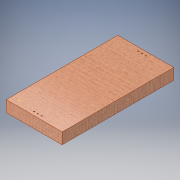
# Autodesk Inventor part: nhk19
Saved by Autodesk Inventor 2019 (Build 230136000, 136)
## iProperties
Created: 2022-02-15
Part Number: nhk19
Material: 木材 (オーク)
Document SubType Name: Sheet Metal
Designer: yuta
Density: 0.76 g/cm^3
Sheet Metal Rule: Default_mm
Appearance: ホワイト オーク材 - ナチュラル 標準の光沢
Author: yuta
Autodesk Inventor part; units mm, degrees
ref_plane "YZ Plane" through (0, 0, 0) normal (1, 0, 0) x (0, 1, 0)
ref_plane "XZ Plane" through (0, 0, 0) normal (0, 1, 0) x (-1, 0, 0)
ref_plane "XY Plane" through (0, 0, 0) normal (0, 0, 1) x (1, 0, 0)
sketch "スケッチ1" plane through (0, 0, 0) normal (0, 1, 0) x (-1, 0, 0)
  line L0 (18.8927, 15.7544) -> (-131.1073, 15.7544)
  line L1 (-131.1073, 15.7544) -> (-131.1073, -284.2456)
  line L2 (-131.1073, -284.2456) -> (18.8927, -284.2456)
  line L3 (18.8927, -284.2456) -> (18.8927, 15.7544)
  point P0 (0, 0)
  dimension "d0" = 150
  dimension "d1" = 300
  constraints: 8 end point, 2 parallel, 1 horizontal, 1 perpendicular
  measures "d0" distance of L2.end L1.end
  measures "d1" distance of L1.end L0.end
extrude "押し出し1" add sketch "スケッチ1" along normal blind 30
sketch "スケッチ2" plane through (0, 30, 0) normal (0, 1, 0) x (1, 0, 0)
  point P0 (0, 0)
sketch "スケッチ3" plane through (0, 30, 0) normal (0, 1, 0) x (1, 0, 0)
  circle A0 centre (56.1073, -5.7544) radius 1.5
  line L0 (-18.8927, 284.2456) -> (-18.8927, -15.7544) projected
  line L1 (-18.8927, -15.7544) -> (131.1073, -15.7544) projected
  circle A1 centre (46.1073, -5.7544) radius 1.5
  circle A2 centre (66.1073, -5.7544) radius 1.5
  point P0 (0, 0)
  dimension "d4" = 3
  dimension "d5" = 75
  dimension "d6" = 10
  dimension "d7" = 3
  dimension "d8" = 3
  dimension "d9" = 10
  dimension "d10" = 10
  constraints: 3 centre point
  measures "d4" diameter of A0
  measures "d5" distance from line of L0 A0.centre
  measures "d6" distance from line of L1 A0.centre
  measures "d7" diameter of A1
  measures "d8" diameter of A2
  measures "d9" distance of A1.centre A0.centre
  measures "d10" distance of A2.centre A0.centre
sketch "スケッチ4" plane through (0, 30, 0) normal (0, 1, 0) x (1, 0, 0)
  circle A0 centre (56.1073, 274.2456) radius 1.5
  line L0 (131.1073, -15.7544) -> (131.1073, 284.2456) projected
  line L1 (131.1073, 284.2456) -> (-18.8927, 284.2456) projected
  circle A1 centre (46.1073, 274.2456) radius 1.5
  circle A2 centre (66.1073, 274.2456) radius 1.5
  point P0 (0, 0)
  dimension "d11" = 3
  dimension "d12" = 75
  dimension "d13" = 10
  dimension "d14" = 3
  dimension "d15" = 3
  dimension "d16" = 10
  dimension "d17" = 10
  constraints: 3 centre point
  measures "d11" diameter of A0
  measures "d12" distance from line of L0 A0.centre
  measures "d13" distance from line of L1 A0.centre
  measures "d14" diameter of A1
  measures "d15" diameter of A2
  measures "d16" distance of A0.centre A1.centre
  measures "d17" distance of A0.centre A2.centre
hole "穴1" at (46.1073, 30, 5.7544) at (56.1073, 30, 5.7544) at (66.1073, 30, 5.7544) direction (0, -1, 0) diameter 3 depth 30
hole "穴2" at (66.1073, 30, -274.2456) at (56.1073, 30, -274.2456) at (46.1073, 30, -274.2456) direction (0, -1, 0) diameter 3 depth 30
equation "\"BendRadius\" = Thickness"
equation "\"BendReliefWidth\" = Thickness"
equation "\"BendReliefDepth\" = 0.5 * Thickness"
equation "\"CornerReliefSize\" = 4 * Thickness"
equation "\"MinimumRemnant\" = 2 * Thickness"
equation "\"TransitionRadius\" = BendRadius"
equation "\"JacobiRadiusSize\" = BendRadius"
equation "\"GapSize\" = Thickness"
equation "\"Thickness\" = 0.5"
